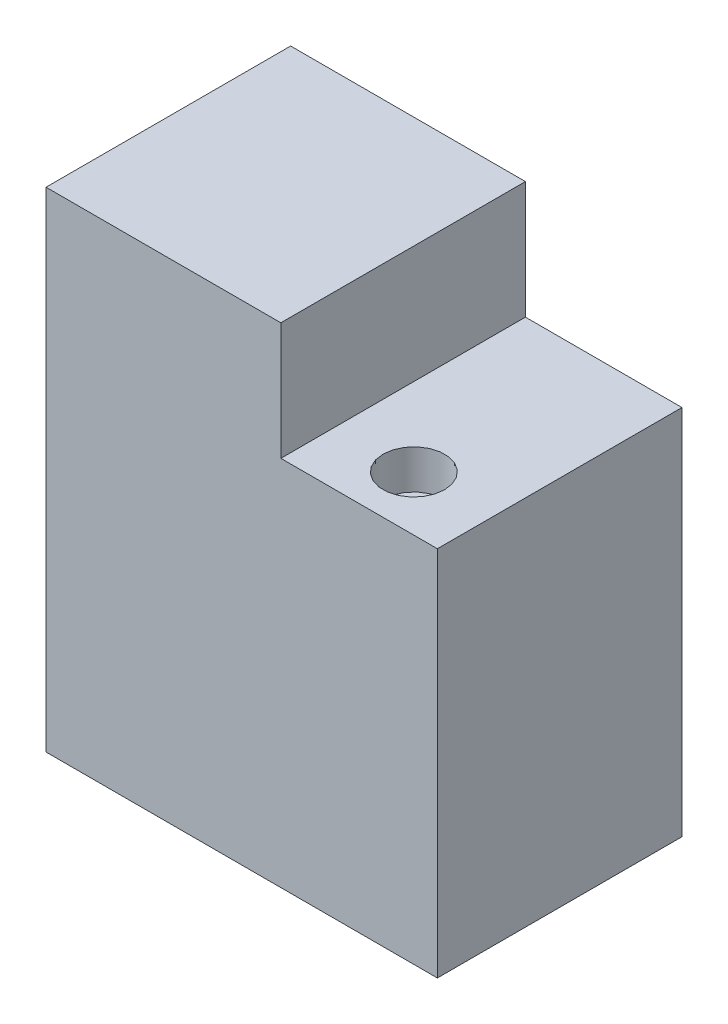
# Autodesk Inventor part: Meal inside front
Saved by Autodesk Inventor 2021 (Build 250183000, 183)
## iProperties
Created: 2020-11-30
Part Number: Meal inside front
Material: Generic
Document SubType Name: Modeling
Designer: deli
Density: 1 g/cm^3
Appearance: Default
Author: deli
Autodesk Inventor part; units mm, degrees
ref_plane "YZ Plane" through (0, 0, 0) normal (1, 0, 0) x (0, 1, 0)
ref_plane "XZ Plane" through (0, 0, 0) normal (0, 1, 0) x (-1, 0, 0)
ref_plane "XY Plane" through (0, 0, 0) normal (0, 0, 1) x (1, 0, 0)
sketch "Sketch1" plane through (0, 0, 0) normal (1, 0, 0) x (0, 1, 0)
  line L0 (36.9572, 50.7029) -> (5.2072, 50.7029)
  line L1 (5.2072, 50.7029) -> (5.2072, 34.8279)
  line L2 (5.2072, 34.8279) -> (36.9572, 34.8279)
  line L3 (36.9572, 34.8279) -> (36.9572, 50.7029)
  point P0 (0, 0)
  dimension "d0" = 31.75
  dimension "d1" = 15.875
  constraints: 8 end point, 2 parallel, 1 horizontal, 1 perpendicular
  measures "d0" distance of L2.end L1.end
  measures "d1" distance of L1.end L0.end
extrude "Extrusion1" add sketch "Sketch1" along normal blind 25.4
sketch "Sketch2" plane through (0, 36.9572, 50.7029) normal (0, 1, 0) x (1, 0, 0)
  line L0 (25.4, 0) -> (25.4, 15.875) projected
  line L1 (0, 0) -> (25.4, 0) projected
  line L2 (25.4, 15.875) -> (15.24, 15.875)
  line L3 (15.24, 15.875) -> (15.24, 0)
  line L4 (15.24, 0) -> (25.4, 0)
  line L5 (25.4, 0) -> (25.4, 15.875)
  point P0 (0, 50.7029)
  dimension "d4" = 10.16
  constraints: 8 end point, 2 parallel, 1 horizontal, 1 perpendicular, 1 point on line
  measures "d4" distance of L4.end L3.end
extrude "Extrusion2" cut sketch "Sketch2" against normal blind 7.62
sketch "Sketch3" plane through (0, 29.3372, 50.7029) normal (0, 1, 0) x (1, 0, 0)
  line L0 (15.24, 0) -> (15.24, 15.875) projected
  line L1 (25.4, 0) -> (15.24, 0) projected
  line L2 (25.4, 15.875) -> (25.4, 0) projected
  line L3 (15.24, 15.875) -> (25.4, 15.875) projected
  circle A0 centre (20.32, 3.5522) radius 2
  point P0 (0, 50.7029)
  dimension "d7" = 4
  dimension "d8" = 5.08
  dimension "d9" = 3.5522
  constraints: 1 centre point
  measures "d7" diameter of A0
  measures "d8" distance from line of L2 A0.centre
  measures "d9" distance from line of L1 A0.centre
extrude "Extrusion3" cut sketch "Sketch3" against normal blind 2.54 contours A0
sketch "Sketch4" plane through (0, 5.2072, 34.8279) normal (0, 0, -1) x (-1, 0, 0)
  circle A0 centre (-10.16, 25.7302) radius 2 projected
  point P0 (0, -5.2072)
extrude "Extrusion4" cut sketch "Sketch4" against normal blind 6.35
body "Solid1"
